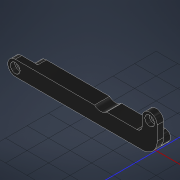
# Autodesk Inventor part: Door_Lever
Saved by Autodesk Inventor 2022.2 (Build 262287010, 287A)
## iProperties
Created: 2022-01-24
Part Number: Door_Lever
Material: ABS-Kunststoff
Document SubType Name: Modeling
Designer: sleib
Density: 1.06 g/cm^3
Appearance: Glatt - Schwarz
Author: sleib
Autodesk Inventor part; units mm, degrees
ref_plane "YZ Plane" through (0, 0, 0) normal (1, 0, 0) x (0, 1, 0)
ref_plane "XZ Plane" through (0, 0, 0) normal (0, 1, 0) x (-1, 0, 0)
ref_plane "XY Plane" through (0, 0, 0) normal (0, 0, 1) x (1, 0, 0)
sketch "Skizze1" plane through (0, 0, 0) normal (0, 0, 1) x (1, 0, 0)
  circle A0 centre (0, 0) radius 2.5
  line L0 (-7, 0) -> (-7, -8)
  line L1 (7, 0) -> (7, -13)
  arc A1 (7, 0) -> (-7, 0) centre (0, 0) ccw
  circle A2 centre (-125, -20) radius 2.5
  line L2 (-125, -13) -> (-12, -13)
  arc A3 (-125, -13) -> (-125, -27) centre (-125, -20) ccw
  line L3 (-7, -27) -> (-125, -27)
  arc A4 (-7, -27) -> (7, -13) centre (-7, -13) ccw
  arc A5 (-12, -13) -> (-7, -8) centre (-12, -8) ccw
  line L4 (-125, -20) -> (0, 0) construction
  circle A6 centre (-45.6749, -7.308) radius 8
  line L5 (-12, -13) -> (0.4833, -13)
  circle A7 centre (-125, -20) radius 7 construction
  arc A8 (-110, -13) -> (-110, -27) centre (-110, -20) ccw
  arc A9 (4.6407, -20.7778) -> (0.4833, -13) centre (0.4833, -18) ccw
  point P0 (-7, -13)
  point P1 (7, -27)
  point P2 (-127.0657, -26.6883)
  point P3 (-40.0535, -13)
  point P4 (-51.2964, -13)
  dimension "d0" = 5
  dimension "d14" = 125
  dimension "d30" = 7
  dimension "d31" = 20
  dimension "d32" = 14
  dimension "d33" = 5
  dimension "d34" = 80.334
  dimension "d37" = 16
  dimension "d47" = 1
  dimension "d48" = 5
  constraints: 14 point on circle, 13 tangent, 12 end point, 10 centre point, 7 point on line, 3 horizontal, 2 coincident, 2 concentric, 2 equal radius, 2 vertical
  measures "d0" diameter of A0
  measures "d14" horizontal distance of point (0, 0) A2.centre
  measures "d30" radius of A1
  measures "d31" vertical distance of point (0, 0) A2.centre
  measures "d32" radius of A4
  measures "d33" radius of A5
  measures "d34" distance of A6.centre A2.centre
  measures "d37" diameter of A6
  measures "d48" radius of A9
extrude "Extrusion1" add sketch "Skizze1" along normal blind 6 contours A1 L1 A4 A9 L5 A5 L0 | L5 A9 A4 L3 A8 L2 A6 | A6 L2 | A8 L3 A3 L2 picked at (-47.0836, -13.3669)
extrude "Extrusion2" cut sketch "Skizze1" along normal through all contours A6 L2 picked at (-47.0836, -13.3669)
extrude "Extrusion3" add sketch "Skizze1" against normal blind 8 contours L5 A9 A4 L3 A8 L2 A6
sketch "Skizze2" plane through (0, 0, 6) normal (0, 0, 1) x (1, 0, 0)
  circle A0 centre (-125, -20) radius 2.5 projected
  circle A1 centre (0, 0) radius 2.5 projected
  constraints: 2 coincident
hole "Bohrung1" at (-125, -20, 6) at (0, 0, 6) direction (0, 0, -1) diameter 5.3 end through all counterbore diameter 9 counterbore depth 4 clearance for "Inbusschraube DIN EN ISO 4762" size "M5" standard "DIN"
